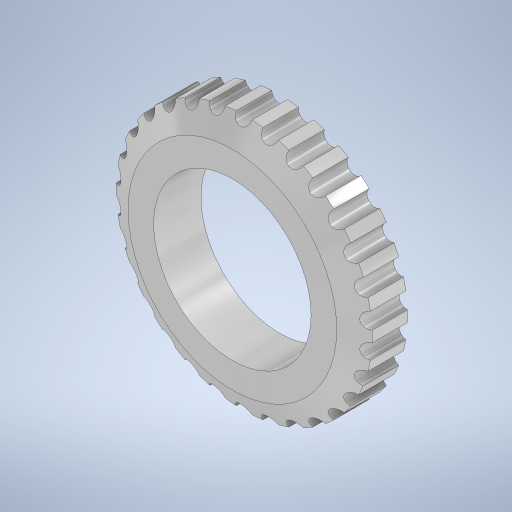
# Autodesk Inventor part: 2.5mm jack nut
Saved by Autodesk Inventor 2024 (Build 280153000, 153)
## iProperties
Created: 2025-09-13
Part Number: 2.5mm jack nut
Material: Generic
Document SubType Name: Modeling
Designer: Login
Density: 1 g/cm^3
Appearance: Default
Author: Login
Autodesk Inventor part; units mm, degrees
ref_plane "YZ Plane" through (0, 0, 0) normal (1, 0, 0) x (0, 1, 0)
ref_plane "XZ Plane" through (0, 0, 0) normal (0, 1, 0) x (-1, 0, 0)
ref_plane "XY Plane" through (0, 0, 0) normal (0, 0, 1) x (1, 0, 0)
sketch "Sketch1" plane through (0, 0, 0) normal (0, 0, 1) x (1, 0, 0)
  circle A0 centre (0, 0) radius 2
  circle A1 centre (0, 0) radius 3.25
  dimension "d0" = 4
  dimension "d1" = 6.5
  constraints: 2 centre point, 2 coincident
  measures "d0" diameter of A0
  measures "d1" diameter of A1
extrude "Extrusion1" add sketch "Sketch1" along normal blind 1.2
chamfer "Chamfer1" distance 0.6 distance2 0.3 1 edges at (-3.25, 0, 1.2) measured on face at (2.7825, -0.4188, 1.2)
sketch "Sketch2" plane through (0, 0, 1.2) normal (0, 0, 1) x (1, 0, 0)
  circle A0 centre (0, 0) radius 3.25 projected
  circle A1 centre (0, 3.25) radius 0.2
  point P0 (-0.1999, 3.2438)
  point P1 (0.1999, 3.2438)
  dimension "d7" = 0.4
  dimension "d8" = 0
  constraints: 1 centre point, 2 other
  measures "d7" diameter of A1
  measures "d8" horizontal distance of point (0, 0) A1.centre
extrude "Extrusion2" cut sketch "Sketch2" against normal through all contours A1 A0 picked at (0.0079, 3.1833)
pattern_circular "Circular Pattern1" count 30 over 360 about axis through (0, 0, 0) along (0, 0, 1) of "Extrusion2"
body "Solid1"
